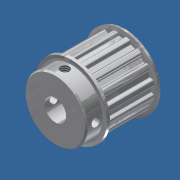
# Autodesk Inventor part: Synchrone Riemenscheibe T5 - Z16 -16mm
Saved by Autodesk Inventor 2016 (Build 200138000, 138)
## iProperties
Created: 2015-01-06
Part Number: Synchrone Riemenscheibe T5 - Z16 -16mm
Material: Aluminium 6061
Document SubType Name: Modeling
Designer: 4ndreas
Density: 2.7 g/cm^3
Appearance: Aluminium - flach
Mass: 25.7609 g
Surface Area: 43.5713 cm^2
Volume: 9.54106 cm^3
CustomPartVersion: 1
Author: 4ndreas
Autodesk Inventor part; units mm, degrees
ref_plane "YZ Plane" through (0, 0, 0) normal (1, 0, 0) x (0, 1, 0)
ref_plane "XZ Plane" through (0, 0, 0) normal (0, 1, 0) x (-1, 0, 0)
ref_plane "XY Plane" through (0, 0, 0) normal (0, 0, 1) x (1, 0, 0)
sketch "Riemenscheibenskizze" plane through (0, 0, 0) normal (0, 0, 1) x (1, 0, 0)
  circle A0 centre (0, 0) radius 12.7324 construction
  circle A1 centre (0, 0) radius 12.2324
  circle A2 centre (0, 0) radius 10.9824
  line L0 (-1.4431, 12.147) -> (-0.9, 10.9824)
  line L1 (-0.9, 10.9824) -> (0.9, 10.9824)
  line L2 (0.9, 10.9824) -> (1.4431, 12.147)
  line L3 (0, 0) -> (0, 12.2324) construction
  point P0 (0, 10.9824)
  dimension "d0" = 25.4648
  dimension "d1" = 0.5
  dimension "d2" = 1.25
  dimension "d3" = 50
  dimension "d4" = 1.8
  constraints: 8 end point, 3 coincident, 3 point on circle, 2 centre point, 1 horizontal, 1 midpoint, 1 point on line, 1 vertical, 1 vertical alignment, 3 other
  measures "d0" diameter of A0
  measures "d1" radial gap between concentric circles of A0 A1
  measures "d3" angle of L2 L0
  measures "d4" distance of L0.end L1.end
extrude "Grundkörper" add sketch "Riemenscheibenskizze" along normal mid plane 17.5 contours A2 | A1 L0 L1 L2 | L2 L1 L0 A1
extrude "Zahn" cut sketch "Riemenscheibenskizze" along normal through all both and the other way through all contours L2 L1 L0 A1 picked at (0, 11.8094)
fillet "Fillet" radius 0.4 2 edges at (0.9, 10.9824, 0) (-0.9, 10.9824, 0)
fillet "Fillet" radius 0.6 4 edges at (-1.4431, 12.147, 4.375) (-1.4431, 12.147, -4.375) (1.4431, 12.147, 4.375) (1.4431, 12.147, -4.375)
pattern_circular "Zähne" count 16 over 360 about axis through (0, 0, -10) along (0, 0, 1) of "Zahn", "Fillet"
pulley flange "Flansch links" diameter 24.4648 height 1.2 thickness 1 bend angle 10 centre (0, 0, -8.75) toward (0, 0, -1)
pulley flange "Flansch rechts" diameter 24.4648 height 1.2 thickness 1 bend angle 10 centre (0, 0, 8.75) toward (0, 0, 1)
sketch "Skizze2" plane through (0, 0, 9.75) normal (0, 0, 1) x (1, 0, 0)
  circle A0 centre (0, 0) radius 15.4155
  circle A1 centre (0, 0) radius 11.5
  dimension "d17" = 23
  constraints: 2 centre point, 1 coincident
  measures "d17" diameter of A1
extrude "Extrusion3" add sketch "Skizze2" along normal blind 6 contours A1
chamfer "Fase1" distance 0.5 angle 45 1 edges at (-11.5, 0, 15.75)
sketch "Skizze3" plane through (0, 0, 15.75) normal (0, 0, 1) x (1, 0, 0)
  circle A0 centre (0, 0) radius 11 projected
hole "Bohrung1" at (0, 0, 15.75) direction (0, 0, -1) diameter 8 end through all
sketch "Skizze4" plane through (0, 0, 15.75) normal (0, 0, 1) x (1, 0, 0)
  line L0 (0, 0) -> (9.2088, 0)
  constraints: 2 end point, 1 horizontal
ref_plane "Arbeitsebene2" through (0, 0, -30.1079) normal (1, 0, 0) x (0, 0, 1)
ref_plane "Arbeitsebene1" through (0, 0, 15.75) normal (0, -1, 0) x (1, 0, 0)
sketch "Skizze5" plane through (0, 0, -30.1079) normal (1, 0, 0) x (0, 0, 1)
  line L0 (21.3579, -10.9824) -> (21.3579, -12.2324) projected
  arc A0 (21.3427, -12.406) -> (21.3579, -12.2324) centre (20.3579, -12.2324) ccw projected
  line L1 (21.3427, -12.406) -> (21.1617, -13.4324) projected
  line L2 (21.1617, -13.4324) -> (20.1769, -13.2587) projected
  line L3 (20.1769, -13.2587) -> (20.3579, -12.2324) projected
  line L4 (20.3579, -12.2324) -> (20.3579, -4) projected
  line L5 (20.3579, -4) -> (45.8579, -4) projected
  line L6 (45.8579, -4) -> (45.8579, -11) projected
  line L7 (45.8579, -11) -> (45.3579, -11.5) projected
  line L8 (45.3579, -11.5) -> (39.8579, -11.5) projected
  line L9 (39.8579, -11.5) -> (39.8579, -12.2324) projected
  line L10 (39.8579, -12.2324) -> (40.0389, -13.2587) projected
  line L11 (40.0389, -13.2587) -> (39.0541, -13.4324) projected
  line L12 (39.0541, -13.4324) -> (38.8731, -12.406) projected
  arc A1 (38.8579, -12.2324) -> (38.8731, -12.406) centre (39.8579, -12.2324) ccw projected
  line L13 (38.8579, -12.2324) -> (38.8579, -10.9824) projected
  line L14 (38.8579, -10.9824) -> (21.3579, -10.9824) projected
  line L15 (21.3579, 12.2324) -> (21.3579, 10.9824) projected
  line L16 (21.3579, 10.9824) -> (38.8579, 10.9824) projected
  line L17 (38.8579, 10.9824) -> (38.8579, 12.2324) projected
  arc A2 (38.8731, 12.406) -> (38.8579, 12.2324) centre (39.8579, 12.2324) ccw projected
  line L18 (38.8731, 12.406) -> (39.0541, 13.4324) projected
  line L19 (39.0541, 13.4324) -> (40.0389, 13.2587) projected
  line L20 (40.0389, 13.2587) -> (39.8579, 12.2324) projected
  line L21 (39.8579, 12.2324) -> (39.8579, 11.5) projected
  line L22 (39.8579, 11.5) -> (45.3579, 11.5) projected
  line L23 (45.3579, 11.5) -> (45.8579, 11) projected
  line L24 (45.8579, 11) -> (45.8579, 4) projected
  line L25 (45.8579, 4) -> (20.3579, 4) projected
  line L26 (20.3579, 4) -> (20.3579, 12.2324) projected
  line L27 (20.3579, 12.2324) -> (20.1769, 13.2587) projected
  line L28 (20.1769, 13.2587) -> (21.1617, 13.4324) projected
  line L29 (21.1617, 13.4324) -> (21.3427, 12.406) projected
  arc A3 (21.3579, 12.2324) -> (21.3427, 12.406) centre (20.3579, 12.2324) ccw projected
  line L30 (45.8579, 4) -> (45.8579, -4)
  circle A4 centre (42.3579, 0) radius 1.6
  line L31 (21.3579, -10.9824) -> (21.3579, -12.2324) projected
  arc A5 (21.3427, -12.406) -> (21.3579, -12.2324) centre (20.3579, -12.2324) ccw projected
  line L32 (21.3427, -12.406) -> (21.1617, -13.4324) projected
  line L33 (21.1617, -13.4324) -> (20.1769, -13.2587) projected
  line L34 (20.1769, -13.2587) -> (20.3579, -12.2324) projected
  line L35 (20.3579, -12.2324) -> (20.3579, -4) projected
  line L36 (20.3579, -4) -> (45.8579, -4) projected
  line L37 (45.8579, -4) -> (45.8579, -11) projected
  line L38 (45.8579, -11) -> (45.3579, -11.5) projected
  line L39 (45.3579, -11.5) -> (39.8579, -11.5) projected
  line L40 (39.8579, -11.5) -> (39.8579, -12.2324) projected
  line L41 (39.8579, -12.2324) -> (40.0389, -13.2587) projected
  line L42 (40.0389, -13.2587) -> (39.0541, -13.4324) projected
  line L43 (39.0541, -13.4324) -> (38.8731, -12.406) projected
  arc A6 (38.8579, -12.2324) -> (38.8731, -12.406) centre (39.8579, -12.2324) ccw projected
  line L44 (38.8579, -12.2324) -> (38.8579, -10.9824) projected
  line L45 (38.8579, -10.9824) -> (21.3579, -10.9824) projected
  line L46 (21.3579, 12.2324) -> (21.3579, 10.9824) projected
  line L47 (21.3579, 10.9824) -> (38.8579, 10.9824) projected
  line L48 (38.8579, 10.9824) -> (38.8579, 12.2324) projected
  arc A7 (38.8731, 12.406) -> (38.8579, 12.2324) centre (39.8579, 12.2324) ccw projected
  line L49 (38.8731, 12.406) -> (39.0541, 13.4324) projected
  line L50 (39.0541, 13.4324) -> (40.0389, 13.2587) projected
  line L51 (40.0389, 13.2587) -> (39.8579, 12.2324) projected
  line L52 (39.8579, 12.2324) -> (39.8579, 11.5) projected
  line L53 (39.8579, 11.5) -> (45.3579, 11.5) projected
  line L54 (45.3579, 11.5) -> (45.8579, 11) projected
  line L55 (45.8579, 11) -> (45.8579, 4) projected
  line L56 (45.8579, 4) -> (20.3579, 4) projected
  line L57 (20.3579, 4) -> (20.3579, 12.2324) projected
  line L58 (20.3579, 12.2324) -> (20.1769, 13.2587) projected
  line L59 (20.1769, 13.2587) -> (21.1617, 13.4324) projected
  line L60 (21.1617, 13.4324) -> (21.3427, 12.406) projected
  arc A8 (21.3579, 12.2324) -> (21.3427, 12.406) centre (20.3579, 12.2324) ccw projected
  line L61 (15.0407, 0) -> (50.9941, 0) projected
  point P0 (30.1079, 0)
  dimension "d32" = 3.2
  dimension "d33" = 3.5
  constraints: 2 end point, 1 centre point, 1 point on line, 1 vertical
  measures "d32" diameter of A4
  measures "d33" distance from line of A4.centre L30
extrude "Extrusion4" cut sketch "Skizze5" along normal through all both and the other way through all contours L61 A4 | A4 L61
sketch "Skizze6" plane through (0, 0, 15.75) normal (0, -1, 0) x (1, 0, 0)
  line L0 (-18.8054, -3.5) -> (18.8054, -3.5) projected
  line L1 (0, -30.8172) -> (0, 5.1362) projected
  point P0 (0, -15.75)
  point P1 (0, -3.5)
  constraints: 1 midpoint, 1 point on line
hole "Bohrung2" at (0, 0, 12.25) direction (0, 1, 0) diameter 3.242 end through all thread size "M4x0.7" class "6H" standard "ANSI Metric M Profile"
equation "\"d1\" = da_a"
equation "\"d2\" = da_hg"
equation "\"d3\" = 2 * da_fi"
equation "\"d4\" = da_bw"
equation "\"d5\" = da_bf"
equation "\"d7\" = da_bf"
equation "\"d9\" = da_rb"
equation "\"d10\" = da_rt"
equation "\"da_pb\" = 5"
equation "\"da_fi\" = 25deg"
equation "\"da_hg\" = 1.25"
equation "\"da_bw\" = 1.8"
equation "\"da_rb\" = 0.4"
equation "\"da_rt\" = 0.6"
equation "\"da_a\" = 0.5"
equation "\"da_bf\" = 17.5"
equation "\"da_wf\" = 1"
equation "\"da_hf\" = 1.2"
body "Solid1"
